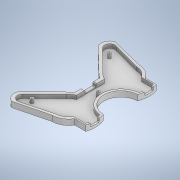
# Autodesk Inventor part: mando_inf
Saved by Autodesk Inventor 2021 (Build 250183000, 183)
## iProperties
Created: 2022-02-28
Part Number: mando_inf
Material: Genérico
Document SubType Name: Modeling
Designer: Joaquín
Density: 1 g/cm^3
Appearance: Valor por defecto
Author: Joaquín
Autodesk Inventor part; units mm, degrees
ref_plane "YZ Plane" through (0, 0, 0) normal (1, 0, 0) x (0, 1, 0)
ref_plane "XZ Plane" through (0, 0, 0) normal (0, 1, 0) x (-1, 0, 0)
ref_plane "XY Plane" through (0, 0, 0) normal (0, 0, 1) x (1, 0, 0)
sketch "Boceto1" plane through (0, 0, 0) normal (0, 1, 0) x (-1, 0, 0)
  line L0 (16, -33) -> (103.2837, -54.9444)
  line L1 (38.5, 50.9711) -> (38.5, 119.0289)
  line L2 (-22.9711, -10.5) -> (-52.9711, -10.5)
  arc A0 (-22.9711, -10.5) -> (16, -33) centre (16, 12) ccw
  arc A1 (-51.515, 38.5517) -> (-6.5, 85) centre (-52.9711, 85) ccw
  arc A2 (-22.9711, -10.5) -> (16, -33) centre (16, 12) ccw
  arc A3 (-51.515, 38.5517) -> (-52.9711, -10.5) centre (16, 12) ccw
  line L3 (38.5, 50.9711) -> (38.5, 85)
  arc A4 (103.2837, -54.9444) -> (115.3375, -21.0974) centre (95.2119, -33) ccw
  line L4 (115.3375, -21.0974) -> (44.6515, 46.7)
  line L5 (16, 203) -> (103.2837, 224.9444)
  arc A5 (16, 203) -> (-22.9711, 180.5) centre (16, 158) ccw
  line L6 (115.3375, 191.0974) -> (44.6515, 123.3)
  arc A6 (115.3375, 191.0974) -> (103.2837, 224.9444) centre (95.2119, 203) ccw
  arc A7 (16, 203) -> (-22.9711, 180.5) centre (16, 158) ccw
  line L7 (38.5, 119.0289) -> (38.5, 50.9711)
  line L8 (-22.9711, 180.5) -> (-52.9711, 180.5)
  line L9 (38.5, 119.0289) -> (38.5, 85)
  arc A8 (-52.9711, 180.5) -> (-51.515, 131.4483) centre (16, 158) ccw
  arc A9 (-6.5, 85) -> (-51.515, 131.4483) centre (-52.9711, 85) ccw
  arc A10 (-22.9711, -10.5) -> (16, -33) centre (16, 12) ccw
  arc A11 (49.4751, 42.0735) -> (38.5, 50.9711) centre (16, 12) ccw
  arc A12 (38.5, 119.0289) -> (49.4751, 127.9265) centre (16, 158) ccw
  arc A13 (16, 203) -> (-22.9711, 180.5) centre (16, 158) ccw
  circle A14 centre (83.6139, -19.9457) radius 1.5
  circle A15 centre (8.5, 85) radius 1.5
  circle A16 centre (83.6139, 189.9457) radius 1.5
  arc A17 (88.6874, -45.3867) -> (105.0119, -23.002) centre (95.2119, -33) ccw
  arc A18 (105.0119, 193.002) -> (91.4604, 216.488) centre (95.2119, 203) ccw
  arc A19 (-48.2434, 32.7133) -> (-48.2434, 137.2867) centre (-52.9711, 85) ccw
  arc A20 (-48.7329, 177.1284) -> (-48.2434, 137.2867) centre (16, 158) ccw
  arc A21 (-48.2434, 32.7133) -> (-48.7329, -7.1284) centre (16, 12) ccw
  line L10 (-48.7329, -7.1284) -> (-16.2545, -7.1284)
  line L11 (-48.7329, 177.1284) -> (-16.2545, 177.1284)
  line L12 (16, 195.5) -> (91.4604, 216.488)
  line L13 (16, -25.5) -> (88.6874, -45.3867)
  line L14 (39.4427, 41.2693) -> (105.0119, -23.002)
  line L15 (105.0119, 193.002) -> (44.7948, 133.9769)
  line L16 (29.5774, 46.9558) -> (29.5774, 123.0442)
  arc A22 (44.7948, 36.0231) -> (29.5774, 46.9558) centre (16, 12) ccw
  arc A23 (-16.2545, -7.1284) -> (16, -25.5) centre (16, 12) ccw
  arc A24 (29.5774, 123.0442) -> (44.7948, 133.9769) centre (16, 158) ccw
  arc A25 (16, 195.5) -> (-16.2545, 177.1284) centre (16, 158) ccw
  circle A26 centre (83.6139, -19.9457) radius 4.5
  circle A27 centre (8.5, 85) radius 4.5
  circle A28 centre (83.6139, 189.9457) radius 4.5
  point P0 (0, 0)
  dimension "d8" = 9
  dimension "d9" = 9
  dimension "d10" = 9
  constraints: 49 point on circle, 34 end point, 29 centre point, 16 coincident, 3 point on line, 2 horizontal, 2 tangent, 1 midpoint, 1 vertical
  measures "d8" diameter of A26
  measures "d9" diameter of A27
  measures "d10" diameter of A28
extrude "Extrusión1" add sketch "Boceto1" along normal blind 10 contours A0 L2 A3 A1 A9 A8 L8 A5 L5 A6 L6 A12 L1 A11 L4 A4 L0 | A26 | A27 | A28
sketch "Boceto2" plane through (0, 0, 0) normal (0, -1, 0) x (1, 0, 0)
  line L0 (-16, 203) -> (-103.2837, 224.9444)
  line L1 (22.9711, 180.5) -> (52.9711, 180.5)
  arc A0 (22.9711, 180.5) -> (-16, 203) centre (-16, 158) ccw
  arc A1 (22.9711, 180.5) -> (-16, 203) centre (-16, 158) ccw
  arc A2 (51.515, 131.4483) -> (52.9711, 180.5) centre (-16, 158) ccw
  line L2 (-38.5, 119.0289) -> (-38.5, 85)
  arc A3 (-103.2837, 224.9444) -> (-115.3375, 191.0974) centre (-95.2119, 203) ccw
  line L3 (-115.3375, 191.0974) -> (-44.6515, 123.3)
  line L4 (-16, -33) -> (-103.2837, -54.9444)
  arc A4 (-16, -33) -> (22.9711, -10.5) centre (-16, 12) ccw
  line L5 (-115.3375, -21.0974) -> (-44.6515, 46.7)
  arc A5 (-115.3375, -21.0974) -> (-103.2837, -54.9444) centre (-95.2119, -33) ccw
  arc A6 (-16, -33) -> (22.9711, -10.5) centre (-16, 12) ccw
  line L6 (22.9711, -10.5) -> (52.9711, -10.5)
  line L7 (-38.5, 50.9711) -> (-38.5, 85)
  arc A7 (52.9711, -10.5) -> (51.515, 38.5517) centre (-16, 12) ccw
  arc A8 (51.515, 131.4483) -> (52.9711, 180.5) centre (-16, 158) ccw projected
  arc A9 (-38.5, 50.9711) -> (-49.4751, 42.0735) centre (-16, 12) ccw
  arc A10 (-16, -33) -> (22.9711, -10.5) centre (-16, 12) ccw
  arc A11 (22.9711, 180.5) -> (-16, 203) centre (-16, 158) ccw
  arc A12 (-49.4751, 127.9265) -> (-38.5, 119.0289) centre (-16, 158) ccw
  arc A13 (51.515, 131.4483) -> (51.515, 38.5517) centre (52.9711, 85) ccw projected
  arc A14 (51.515, 131.4483) -> (51.515, 38.5517) centre (52.9711, 85) ccw
  point P0 (0, 170)
  constraints: 29 point on circle, 16 end point, 13 centre point, 7 coincident, 2 point on line
extrude "Extrusión2" add sketch "Boceto2" along normal blind 5 contours A0 L1 A2 A13 A7 L6 A4 L4 A5 L5 A9 L7 L2 A12 L3 A3 L0
sketch "Boceto3" plane through (-29.5774, 10, 123.0442) normal (1, 0, 0) x (0, 0, -1)
  line L0 (0, 0) -> (76.0885, 0) projected
  line L1 (38.0442, 0) -> (53.0442, 0)
  line L2 (72.0731, 0) -> (4.0154, 0) projected
  line L3 (38.0442, 0) -> (23.0442, 0)
  line L4 (23.0442, 0) -> (23.0442, -8)
  line L5 (23.0442, -8) -> (53.0442, -8)
  line L6 (53.0442, -8) -> (53.0442, 0)
  point P0 (123.0442, -10)
  point P1 (53.0442, 0)
  point P2 (23.0442, 0)
  dimension "d15" = 15
  dimension "d16" = 15
  dimension "d17" = 8
  constraints: 10 end point, 3 perpendicular, 2 point on line, 1 midpoint
  measures "d15" distance of L1.start L1.end
  measures "d16" distance of L1.start L3.end
  measures "d17" distance of L3.end L4.end
extrude "Extrusión3" cut sketch "Boceto3" against normal blind 15
fillet "Empalme1" radius 2 4 edges at (-34.0387, 2, 100) (-34.0387, 2, 70) (-34.0387, 10, 70) (-34.0387, 10, 100)
sketch "Boceto4" plane through (0, 10, 0) normal (0, 1, 0) x (1, 0, 0)
  line L0 (59.5944, 0) -> (46.2124, 0)
  line L1 (46.2124, 0) -> (46.2124, -23.3919)
  line L2 (46.2124, -23.3919) -> (63.6147, -23.3919)
  line L3 (63.6147, -23.3919) -> (63.6147, 0)
  circle A0 centre (-8.5, -85) radius 1.5 projected
  line L4 (-8.5, -85) -> (35.636, -85)
  line L5 (59.5944, -170) -> (46.2124, -170)
  line L6 (46.2124, -170) -> (46.2124, -146.6081)
  line L7 (46.2124, -146.6081) -> (63.6147, -146.6081)
  line L8 (63.6147, -146.6081) -> (63.6147, -170)
  line L9 (59.5944, -170) -> (63.6147, -170)
  line L10 (63.6147, 0) -> (58.9449, 0)
  point P0 (0, 0)
  constraints: 22 end point, 5 symmetric about line, 4 perpendicular, 3 point on line, 2 horizontal
extrude "Extrusión4" cut sketch "Boceto4" against normal blind 8 contours L10 L3 L2 L1 L0 | L5 L6 L7 L8 L9
fillet "Empalme2" radius 2 8 edges at (53.0901, 2, 146.6081) (52.9869, 2, 170) (52.9869, 10, 170) (53.0901, 10, 146.6081) (53.0901, 2, 23.3919) (52.9869, 2, 0) (52.9869, 10, 0) (53.0901, 10, 23.3919)
